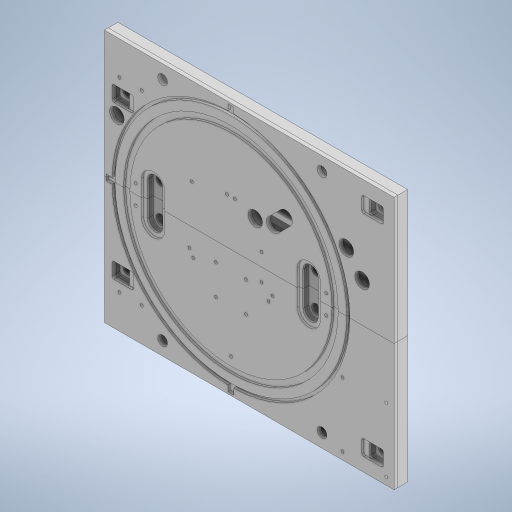
# Autodesk Inventor part: Корпус
Saved by Autodesk Inventor 2024 (Build 280153020, 153B)
## iProperties
Created: 2023-02-24
Part Number: Корпус
Material: Типовые
Document SubType Name: Modeling
Designer: Admin
Density: 1 g/cm^3
Appearance: По умолчанию
Author: Admin
Autodesk Inventor part; units mm, degrees
(part 1 of 3)
ref_plane "YZ Plane" through (0, 0, 0) normal (1, 0, 0) x (0, 1, 0)
ref_plane "XZ Plane" through (0, 0, 0) normal (0, 1, 0) x (-1, 0, 0)
ref_plane "XY Plane" through (0, 0, 0) normal (0, 0, 1) x (1, 0, 0)
sketch "Эскиз1" plane through (0, 0, 0) normal (0, 0, 1) x (1, 0, 0)
  circle A0 centre (0, 0) radius 118.266 construction
  circle A1 centre (0, 0) radius 119.25
  line L0 (-126.25, 126.25) -> (163.75, 126.25)
  line L1 (163.75, 126.25) -> (163.75, -126.25)
  line L2 (163.75, -126.25) -> (-126.25, -126.25)
  line L3 (-126.25, -126.25) -> (-126.25, 126.25)
  circle A2 centre (0, 0) radius 122.25
  line L4 (-3, 122.2132) -> (-3, 128.25)
  line L5 (-3, 128.25) -> (3, 128.25)
  line L6 (3, 128.25) -> (3, 122.2132)
  line L7 (-122.2132, 3) -> (-128.25, 3)
  line L8 (-128.25, 3) -> (-128.25, -3)
  line L9 (-128.25, -3) -> (-122.2132, -3)
  line L10 (3, -122.2132) -> (3, -128.25)
  line L11 (3, -128.25) -> (-3, -128.25)
  line L12 (-3, -128.25) -> (-3, -122.2132)
  line L13 (167.75, 130.25) -> (-130.25, 130.25)
  line L14 (-130.25, 130.25) -> (-130.25, -130.25)
  line L15 (-130.25, -130.25) -> (167.75, -130.25)
  line L16 (167.75, -130.25) -> (167.75, 130.25)
  line L17 (-126.25, 126.25) -> (-126.25, 130.25)
  line L18 (-126.25, -126.25) -> (-126.25, -130.25)
  line L19 (163.75, -126.25) -> (163.75, -130.25)
  line L20 (163.75, 126.25) -> (163.75, 130.25)
  circle A3 centre (0, 0) radius 104
  circle A4 centre (0, 0) radius 110.3675
  circle A5 centre (0, 0) radius 63
  line L21 (-80.25, 126.25) -> (-126.25, 126.25)
  line L22 (-80.25, 101.25) -> (-80.25, 126.25)
  line L23 (-126.25, 126.25) -> (-126.25, 101.25)
  line L24 (-126.25, 101.25) -> (-80.25, 101.25)
  line L25 (-126.25, -126.25) -> (-80.25, -126.25)
  line L26 (-80.25, -101.25) -> (-126.25, -101.25)
  line L27 (-126.25, -101.25) -> (-126.25, -126.25)
  line L28 (-80.25, -126.25) -> (-80.25, -101.25)
  line L29 (-70.25, 121.25) -> (93.75, 121.25) construction
  line L30 (-70.25, 111.25) -> (93.75, 111.25) construction
  circle A6 centre (93.75, 116.25) radius 5
  circle A7 centre (-70.25, 116.25) radius 5
  circle A8 centre (0, 0) radius 55.4255 construction
  line L31 (0, -27.1116) -> (0, -26.4367) construction
  line L32 (0, 0) -> (156.4435, 0) construction
  line L33 (0, 0) -> (156.0708, 16.4588) construction
  line L34 (0, 0) -> (155.7905, -16.4292) construction
  line L35 (-128.25, 0) -> (-119.25, 0)
  line L36 (0, -128.25) -> (0, -119.25)
  line L37 (0, 128.25) -> (0, 119.25)
  line L38 (163.75, 116.25) -> (163.75, 100.25)
  line L39 (163.75, 100.25) -> (163.75, 116.25)
  circle A9 centre (0, -34.641) radius 20.7845 construction
  line L40 (93, -126.25) -> (108, -126.25)
  line L41 (-76, -126.25) -> (-61, -126.25)
  line L42 (14, -6) -> (49, -6) construction
  line L43 (49, -6) -> (49, 6) construction
  line L44 (49, 6) -> (14, 6) construction
  line L45 (14, 6) -> (14, -6) construction
  line L46 (14, -6) -> (49, 6) construction
  line L47 (49, -6) -> (14, 6) construction
  line L48 (36.5689, 0.8398) -> (49, 2.1508) construction
  line L49 (49, 2.1508) -> (48.3707, 8.1177) construction
  line L50 (48.3707, 8.1177) -> (35.9397, 6.8067) construction
  line L51 (35.9397, 6.8067) -> (36.5689, 0.8398) construction
  line L52 (36.5689, 0.8398) -> (48.3707, 8.1177) construction
  line L53 (49, 2.1508) -> (35.9397, 6.8067) construction
  line L54 (35.9397, -6.8067) -> (48.3707, -8.1177) construction
  line L55 (48.3707, -8.1177) -> (49, -2.1508) construction
  line L56 (49, -2.1508) -> (36.5689, -0.8398) construction
  line L57 (36.5689, -0.8398) -> (35.9397, -6.8067) construction
  line L58 (35.9397, -6.8067) -> (49, -2.1508) construction
  line L59 (48.3707, -8.1177) -> (36.5689, -0.8398) construction
  line L60 (14, -11) -> (49, -11)
  line L61 (49, -11) -> (49, 11)
  line L62 (49, 11) -> (14, 11)
  line L63 (19, 11) -> (19, -11)
  line L64 (0, 0) -> (63, 0) construction
  line L65 (34.5, -11) -> (28.5, -11)
  line L66 (28.5, -11) -> (28.5, -16)
  line L67 (28.5, -16) -> (34.5, -16)
  line L68 (34.5, -16) -> (34.5, -11)
  line L69 (28.5, 11) -> (34.5, 11)
  line L70 (34.5, 11) -> (34.5, 16)
  line L71 (34.5, 16) -> (28.5, 16)
  line L72 (28.5, 16) -> (28.5, 11)
  circle A10 centre (31.5, 13.5) radius 1.5
  line L73 (29.9412, 10.8) -> (28.3823, 13.5)
  line L74 (28.3823, 13.5) -> (29.9412, 16.2)
  line L75 (29.9412, 16.2) -> (33.0588, 16.2)
  line L76 (33.0588, 16.2) -> (34.6177, 13.5)
  line L77 (34.6177, 13.5) -> (33.0588, 10.8)
  line L78 (33.0588, 10.8) -> (29.9412, 10.8)
  arc A11 (34.5, 16) -> (49, 11) centre (49, 34.525) ccw
  arc A12 (49, -11) -> (34.5, -16) centre (49, -34.525) ccw
  arc A13 (14, -11) -> (28.5, -16) centre (28.5, 7.525) ccw
  arc A14 (28.5, 16) -> (16.5, 9) centre (28.5, 2.2143) ccw construction
  circle A15 centre (93.75, -116.25) radius 5
  line L79 (-70.25, -111.25) -> (93.75, -111.25) construction
  line L80 (-70.25, -121.25) -> (93.75, -121.25) construction
  circle A16 centre (-70.25, -116.25) radius 5
  circle A17 centre (-117.25, 60.75) radius 7.5
  circle A18 centre (118.75, 60.75) radius 7.5
  line L81 (-117.25, 68.25) -> (118.75, 68.25) construction
  line L82 (118.75, 53.25) -> (-117.25, 53.25) construction
  circle A19 centre (25, 40) radius 7.5
  circle A20 centre (135, 40) radius 7.5
  line L83 (135, 47.5) -> (25, 47.5) construction
  line L84 (135, 32.5) -> (25, 32.5) construction
  line L85 (162.25, -54.75) -> (112.25, -54.75)
  line L86 (112.25, -54.75) -> (112.25, -124.75)
  line L87 (112.25, -124.75) -> (162.25, -124.75)
  line L88 (162.25, -124.75) -> (162.25, -54.75)
  circle A21 centre (159.75, -56.75) radius 1.5
  circle A22 centre (114.75, -56.75) radius 1.5
  circle A23 centre (114.75, -122.75) radius 1.5
  circle A24 centre (159.75, -122.75) radius 1.5
  line L89 (137.25, -89.75) -> (144.5274, -89.75) construction
  line L90 (144.5274, -89.75) -> (137.25, -89.75) construction
  line L91 (137.25, -89.75) -> (137.25, -87.3142) construction
  circle A25 centre (-47.6314, -27.5) radius 8 construction
  circle A26 centre (0, 55) radius 8 construction
  circle A27 centre (-47.6314, -27.5) radius 2.5
  line L92 (54.5596, -31.5) -> (0, 63) construction
  line L93 (0, 63) -> (-54.5596, -31.5) construction
  line L94 (-54.5596, -31.5) -> (54.5596, -31.5) construction
  line L95 (-35.6542, -29.2452) -> (-49.5106, -37.2452)
  line L96 (-49.5106, -37.2452) -> (-57.0106, -24.2548)
  line L97 (-57.0106, -24.2548) -> (-43.1542, -16.2548)
  line L98 (-40.4221, -16.9869) -> (-34.9221, -26.5131)
  line L99 (-33.9221, -28.2452) -> (-57.0106, -24.2548) construction
  line L100 (-49.5106, -37.2452) -> (-41.4221, -15.2548) construction
  line L101 (-47.6314, -27.5) -> (0, 0) construction
  circle A28 centre (-42.7032, -20.0359) radius 1.5
  line L102 (0, 0) -> (0, 14.3794) construction
  circle A29 centre (-38.7032, -26.9641) radius 1.5
  line L103 (21.15, -13.491) -> (-21.15, -13.491)
  line L104 (-21.15, -13.491) -> (-21.15, -55.791)
  line L105 (-21.15, -55.791) -> (21.15, -55.791)
  line L106 (21.15, -55.791) -> (21.15, -13.491)
  line L107 (21.15, -13.491) -> (-21.15, -55.791) construction
  line L108 (-21.15, -13.491) -> (21.15, -55.791) construction
  circle A30 centre (15.5, -50.141) radius 1.5
  line L109 (0, -34.641) -> (0, -31.0481)
  line L110 (0, -34.641) -> (5.9719, -34.641)
  circle A31 centre (-15.5, -50.141) radius 1.5
  circle A32 centre (-15.5, -19.141) radius 1.5
  circle A33 centre (15.5, -19.141) radius 1.5
  line L111 (16.5, -13.491) -> (21.15, -18.141)
  line L112 (-16.5, -13.491) -> (-21.15, -18.141)
  line L113 (14, 11) -> (14, -11)
  line L114 (19, -11) -> (19, 11)
  line L115 (-43.1542, -16.2548) -> (-40.4221, -16.9869)
  line L116 (-35.6542, -29.2452) -> (-34.9221, -26.5131)
  line L117 (34.9221, -26.5131) -> (40.4221, -16.9869)
  line L118 (35.6542, -29.2452) -> (34.9221, -26.5131)
  line L119 (49.5106, -37.2452) -> (35.6542, -29.2452)
  line L120 (57.0106, -24.2548) -> (49.5106, -37.2452)
  line L121 (43.1542, -16.2548) -> (57.0106, -24.2548)
  line L122 (43.1542, -16.2548) -> (40.4221, -16.9869)
  circle A34 centre (42.7032, -20.0359) radius 1.5
  circle A35 centre (38.7032, -26.9641) radius 1.5
  circle A36 centre (47.6314, -27.5) radius 2.5
  circle A37 centre (47.6314, -27.5) radius 8 construction
  line L123 (57.0106, -24.2548) -> (33.9221, -28.2452) construction
  line L124 (41.4221, -15.2548) -> (49.5106, -37.2452) construction
  line L125 (5.5, 43.5) -> (-5.5, 43.5)
  line L126 (7.5, 45.5) -> (5.5, 43.5)
  line L127 (7.5, 61.5) -> (7.5, 45.5)
  line L128 (-7.5, 61.5) -> (7.5, 61.5)
  line L129 (-7.5, 45.5) -> (-7.5, 61.5)
  line L130 (-7.5, 45.5) -> (-5.5, 43.5)
  circle A38 centre (-4, 47) radius 1.5
  circle A39 centre (4, 47) radius 1.5
  circle A40 centre (0, 55) radius 2.5
  circle A41 centre (0, 55) radius 8 construction
  line L131 (-7.5, 61.5) -> (7.5, 43.5) construction
  line L132 (-7.5, 43.5) -> (7.5, 61.5) construction
  line L133 (163.75, -116.25) -> (163.75, -100.25)
  line L134 (163.75, -100.25) -> (163.75, -116.25)
  line L135 (-109.3, 75.8921) -> (-114.25, 73.0342)
  line L136 (-114.25, 73.0342) -> (-119.2, 75.8921)
  line L137 (-119.2, 75.8921) -> (-119.2, 81.6079)
  line L138 (-119.2, 81.6079) -> (-114.25, 84.4658)
  line L139 (-114.25, 84.4658) -> (-109.3, 81.6079)
  line L140 (-109.3, 81.6079) -> (-109.3, 75.8921)
  line L141 (-120.25, 70.75) -> (-108.25, 70.75)
  line L142 (-106.25, 72.75) -> (-106.25, 84.75)
  line L143 (-108.25, 86.75) -> (-120.25, 86.75)
  line L144 (-122.25, 84.75) -> (-122.25, 72.75)
  line L145 (-122.25, 70.75) -> (-106.25, 86.75) construction
  line L146 (-106.25, 70.75) -> (-122.25, 86.75) construction
  arc A42 (-120.25, 86.75) -> (-122.25, 84.75) centre (-120.25, 84.75) ccw
  arc A43 (-108.25, 70.75) -> (-106.25, 72.75) centre (-108.25, 72.75) ccw
  arc A44 (-106.25, 84.75) -> (-108.25, 86.75) centre (-108.25, 84.75) ccw
  arc A45 (-122.25, 72.75) -> (-120.25, 70.75) centre (-120.25, 72.75) ccw
  line L147 (-109.3, -75.8921) -> (-114.25, -73.0342)
  line L148 (-114.25, -73.0342) -> (-119.2, -75.8921)
  line L149 (-119.2, -75.8921) -> (-119.2, -81.6079)
  line L150 (-119.2, -81.6079) -> (-114.25, -84.4658)
  line L151 (-114.25, -84.4658) -> (-109.3, -81.6079)
  line L152 (-109.3, -81.6079) -> (-109.3, -75.8921)
  line L153 (-120.25, -70.75) -> (-108.25, -70.75)
  line L154 (-106.25, -72.75) -> (-106.25, -84.75)
  line L155 (-108.25, -86.75) -> (-120.25, -86.75)
  line L156 (-122.25, -84.75) -> (-122.25, -72.75)
  line L157 (-122.25, -70.75) -> (-106.25, -86.75) construction
  line L158 (-106.25, -70.75) -> (-122.25, -86.75) construction
  arc A46 (-122.25, -84.75) -> (-120.25, -86.75) centre (-120.25, -84.75) ccw
  arc A47 (-106.25, -72.75) -> (-108.25, -70.75) centre (-108.25, -72.75) ccw
  arc A48 (-108.25, -86.75) -> (-106.25, -84.75) centre (-108.25, -84.75) ccw
  arc A49 (-120.25, -70.75) -> (-122.25, -72.75) centre (-120.25, -72.75) ccw
  line L159 (-126.25, 101.25) -> (-80.25, 101.25)
  circle A50 centre (-114.75, 95.75) radius 1.5
  circle A51 centre (-91.75, 95.75) radius 1.5
  line L160 (-112.05, 97.3088) -> (-112.05, 94.1912)
  line L161 (-112.05, 94.1912) -> (-114.75, 92.6323)
  line L162 (-114.75, 92.6323) -> (-117.45, 94.1912)
  line L163 (-117.45, 94.1912) -> (-117.45, 97.3088)
  line L164 (-117.45, 97.3088) -> (-114.75, 98.8677)
  line L165 (-114.75, 98.8677) -> (-112.05, 97.3088)
  line L166 (-91.75, 98.8677) -> (-89.05, 97.3088)
  line L167 (-89.05, 97.3088) -> (-89.05, 94.1912)
  line L168 (-89.05, 94.1912) -> (-91.75, 92.6323)
  line L169 (-91.75, 92.6323) -> (-94.45, 94.1912)
  line L170 (-94.45, 94.1912) -> (-94.45, 97.3088)
  line L171 (-94.45, 97.3088) -> (-91.75, 98.8677)
  line L172 (-117.5, 91) -> (-112, 91)
  line L173 (-110, 93) -> (-110, 98.5)
  line L174 (-112, 100.5) -> (-117.5, 100.5)
  line L175 (-119.5, 98.5) -> (-119.5, 93)
  line L176 (-119.5, 91) -> (-110, 100.5) construction
  line L177 (-110, 91) -> (-119.5, 100.5) construction
  line L178 (-89, 100.5) -> (-94.5, 100.5)
  line L179 (-96.5, 98.5) -> (-96.5, 93)
  line L180 (-94.5, 91) -> (-89, 91)
  line L181 (-87, 93) -> (-87, 98.5)
  line L182 (-87, 100.5) -> (-96.5, 91) construction
  line L183 (-96.5, 100.5) -> (-87, 91) construction
  arc A52 (-119.5, 93) -> (-117.5, 91) centre (-117.5, 93) ccw
  arc A53 (-117.5, 100.5) -> (-119.5, 98.5) centre (-117.5, 98.5) ccw
  arc A54 (-110, 98.5) -> (-112, 100.5) centre (-112, 98.5) ccw
  arc A55 (-112, 91) -> (-110, 93) centre (-112, 93) ccw
  arc A56 (-96.5, 93) -> (-94.5, 91) centre (-94.5, 93) ccw
  arc A57 (-94.5, 100.5) -> (-96.5, 98.5) centre (-94.5, 98.5) ccw
  arc A58 (-89, 91) -> (-87, 93) centre (-89, 93) ccw
  arc A59 (-87, 98.5) -> (-89, 100.5) centre (-89, 98.5) ccw
  line L184 (-126.25, -101.25) -> (-80.25, -101.25)
  line L185 (-80.25, -101.25) -> (-80.25, -100.25)
  line L186 (-90.25, -90.25) -> (-116.25, -90.25)
  circle A60 centre (-91.75, -95.75) radius 1.5
  line L187 (-91.75, -92.6323) -> (-89.05, -94.1912)
  line L188 (-89.05, -94.1912) -> (-89.05, -97.3088)
  line L189 (-89.05, -97.3088) -> (-91.75, -98.8677)
  line L190 (-91.75, -98.8677) -> (-94.45, -97.3088)
  line L191 (-94.45, -97.3088) -> (-94.45, -94.1912)
  line L192 (-94.45, -94.1912) -> (-91.75, -92.6323)
  line L193 (-94.5, -100.5) -> (-89, -100.5)
  line L194 (-87, -98.5) -> (-87, -93)
  line L195 (-89, -91) -> (-94.5, -91)
  line L196 (-96.5, -93) -> (-96.5, -98.5)
  line L197 (-96.5, -100.5) -> (-87, -91) construction
  line L198 (-87, -100.5) -> (-96.5, -91) construction
  arc A61 (-94.5, -91) -> (-96.5, -93) centre (-94.5, -93) ccw
  arc A62 (-89, -100.5) -> (-87, -98.5) centre (-89, -98.5) ccw
  arc A63 (-96.5, -98.5) -> (-94.5, -100.5) centre (-94.5, -98.5) ccw
  arc A64 (-87, -93) -> (-89, -91) centre (-89, -93) ccw
  line L199 (-117.5, -100.5) -> (-112, -100.5)
  line L200 (-110, -98.5) -> (-110, -93)
  line L201 (-112, -91) -> (-117.5, -91)
  line L202 (-119.5, -93) -> (-119.5, -98.5)
  line L203 (-119.5, -100.5) -> (-110, -91) construction
  line L204 (-110, -100.5) -> (-119.5, -91) construction
  circle A65 centre (-114.75, -95.75) radius 1.5
  line L205 (-112.05, -94.1912) -> (-112.05, -97.3088)
  line L206 (-112.05, -97.3088) -> (-114.75, -98.8677)
  line L207 (-114.75, -98.8677) -> (-117.45, -97.3088)
  line L208 (-117.45, -97.3088) -> (-117.45, -94.1912)
  line L209 (-117.45, -94.1912) -> (-114.75, -92.6323)
  line L210 (-114.75, -92.6323) -> (-112.05, -94.1912)
  line L211 (-126.25, -100.25) -> (-126.25, -101.25)
  arc A66 (-117.5, -91) -> (-119.5, -93) centre (-117.5, -93) ccw
  arc A67 (-110, -93) -> (-112, -91) centre (-112, -93) ccw
  arc A68 (-112, -100.5) -> (-110, -98.5) centre (-112, -98.5) ccw
  arc A69 (-119.5, -98.5) -> (-117.5, -100.5) centre (-117.5, -98.5) ccw
  line L212 (-108.25, 86.75) -> (-102.25, 86.75)
  line L213 (-100.25, 84.75) -> (-100.25, 72.75)
  line L214 (-102.25, 70.75) -> (-108.25, 70.75)
  line L215 (-108.25, 70.75) -> (-108.25, 86.75)
  line L216 (-108.25, -86.75) -> (-102.25, -86.75)
  line L217 (-100.25, -84.75) -> (-100.25, -72.75)
  line L218 (-102.25, -70.75) -> (-108.25, -70.75)
  line L219 (-108.25, -70.75) -> (-108.25, -86.75)
  circle A70 centre (-114.25, 78.75) radius 3
  circle A71 centre (-114.25, -78.75) radius 3
  line L220 (4, 50.1177) -> (6.7, 48.5588)
  line L221 (6.7, 48.5588) -> (6.7, 45.4412)
  line L222 (6.7, 45.4412) -> (4, 43.8823)
  line L223 (4, 43.8823) -> (1.3, 45.4412)
  line L224 (1.3, 45.4412) -> (1.3, 48.5588)
  line L225 (1.3, 48.5588) -> (4, 50.1177)
  line L226 (-7.7, 42.25) -> (7.7, 42.25)
  line L227 (9.7, 44.25) -> (9.7, 49.75)
  line L228 (7.7, 51.75) -> (-7.7, 51.75)
  line L229 (-9.7, 49.75) -> (-9.7, 44.25)
  arc A72 (-7.7, 51.75) -> (-9.7, 49.75) centre (-7.7, 49.75) ccw
  arc A73 (7.7, 42.25) -> (9.7, 44.25) centre (7.7, 44.25) ccw
  arc A74 (-9.7, 44.25) -> (-7.7, 42.25) centre (-7.7, 44.25) ccw
  arc A75 (9.7, 49.75) -> (7.7, 51.75) centre (7.7, 49.75) ccw
  line L230 (0, 42.25) -> (0, 44.9705) construction
  circle A76 centre (-4, 47) radius 1.5
  line L231 (-6.7, 45.4412) -> (-4, 43.8823)
  line L232 (-6.7, 48.5588) -> (-6.7, 45.4412)
  line L233 (-4, 43.8823) -> (-1.3, 45.4412)
  line L234 (-4, 50.1177) -> (-6.7, 48.5588)
  line L235 (-1.3, 45.4412) -> (-1.3, 48.5588)
  line L236 (-1.3, 48.5588) -> (-4, 50.1177)
  line L237 (-42.7032, -16.9182) -> (-40.0032, -18.4771)
  arc A77 (-40.4396, -14.4566) -> (-43.1716, -13.7246) centre (-42.1716, -15.4566) ccw
  line L238 (-36.5896, -21.125) -> (-38.9456, -22.4853) construction
  arc A78 (-40.9668, -32.5434) -> (-38.2348, -33.2754) centre (-39.2348, -31.5434) ccw
  line L239 (-38.2348, -33.2754) -> (-33.4716, -30.5254)
  line L240 (-38.7032, -30.0818) -> (-36.0032, -28.5229)
  arc A79 (-33.4716, -30.5254) -> (-32.7396, -27.7934) centre (-34.4716, -28.7934) ccw
  line L241 (-41.4032, -28.5229) -> (-38.7032, -30.0818)
  line L242 (-36.0032, -28.5229) -> (-36.0032, -25.4053)
  line L243 (-41.4032, -25.4053) -> (-41.4032, -28.5229)
  line L244 (-38.7032, -23.8464) -> (-41.4032, -25.4053)
  line L245 (-36.0032, -25.4053) -> (-38.7032, -23.8464)
  line L246 (-40.0032, -18.4771) -> (-40.0032, -21.5947)
  line L247 (-40.0032, -21.5947) -> (-42.7032, -23.1536)
  line L248 (-42.7032, -23.1536) -> (-45.4032, -21.5947)
  line L249 (-45.4032, -21.5947) -> (-45.4032, -18.4771)
  line L250 (-32.7396, -27.7934) -> (-40.4396, -14.4566)
  line L251 (-48.6668, -19.2066) -> (-40.9668, -32.5434)
  arc A80 (-47.9348, -16.4746) -> (-48.6668, -19.2066) centre (-46.9348, -18.2066) ccw
  line L252 (-43.1716, -13.7246) -> (-47.9348, -16.4746)
  line L253 (-45.4032, -18.4771) -> (-42.7032, -16.9182)
  line L254 (36.0032, -28.5229) -> (36.0032, -25.4053)
  arc A81 (32.7396, -27.7934) -> (33.4716, -30.5254) centre (34.4716, -28.7934) ccw
  line L255 (36.5896, -21.125) -> (38.9456, -22.4853) construction
  arc A82 (48.6668, -19.2066) -> (47.9348, -16.4746) centre (46.9348, -18.2066) ccw
  line L256 (47.9348, -16.4746) -> (43.1716, -13.7246)
  line L257 (45.4032, -18.4771) -> (42.7032, -16.9182)
  arc A83 (43.1716, -13.7246) -> (40.4396, -14.4566) centre (42.1716, -15.4566) ccw
  line L258 (45.4032, -21.5947) -> (45.4032, -18.4771)
  line L259 (42.7032, -16.9182) -> (40.0032, -18.4771)
  line L260 (42.7032, -23.1536) -> (45.4032, -21.5947)
  line L261 (40.0032, -21.5947) -> (42.7032, -23.1536)
  line L262 (40.0032, -18.4771) -> (40.0032, -21.5947)
  line L263 (36.0032, -25.4053) -> (38.7032, -23.8464)
  line L264 (38.7032, -23.8464) -> (41.4032, -25.4053)
  line L265 (41.4032, -25.4053) -> (41.4032, -28.5229)
  line L266 (41.4032, -28.5229) -> (38.7032, -30.0818)
  line L267 (40.4396, -14.4566) -> (32.7396, -27.7934)
  line L268 (40.9668, -32.5434) -> (48.6668, -19.2066)
  arc A84 (38.2348, -33.2754) -> (40.9668, -32.5434) centre (39.2348, -31.5434) ccw
  line L269 (33.4716, -30.5254) -> (38.2348, -33.2754)
  line L270 (38.7032, -30.0818) -> (36.0032, -28.5229)
  line L271 (37.5303, -23.4956) -> (25.475, -16.5355)
  line L272 (24.743, -13.8035) -> (28.3843, -7.4965)
  line L273 (31.1164, -6.7645) -> (43.1716, -13.7246)
  line L274 (43.1716, -13.7246) -> (37.5303, -23.4956)
  line L275 (37.5303, -23.4956) -> (29.3843, -5.7645) construction
  line L276 (23.743, -15.5355) -> (43.1716, -13.7246) construction
  arc A85 (24.743, -13.8035) -> (25.475, -16.5355) centre (26.475, -14.8035) ccw
  arc A86 (31.1164, -6.7645) -> (28.3843, -7.4965) centre (30.1164, -8.4965) ccw
  line L277 (28.75, 8.75) -> (34.25, 8.75)
  line L278 (36.25, 10.75) -> (36.25, 16.25)
  line L279 (34.25, 18.25) -> (28.75, 18.25)
  line L280 (26.75, 16.25) -> (26.75, 10.75)
  line L281 (26.75, 8.75) -> (36.25, 18.25) construction
  line L282 (36.25, 8.75) -> (26.75, 18.25) construction
  arc A87 (28.75, 18.25) -> (26.75, 16.25) centre (28.75, 16.25) ccw
  arc A88 (36.25, 16.25) -> (34.25, 18.25) centre (34.25, 16.25) ccw
  arc A89 (26.75, 10.75) -> (28.75, 8.75) centre (28.75, 10.75) ccw
  arc A90 (34.25, 8.75) -> (36.25, 10.75) centre (34.25, 10.75) ccw
  line L283 (15.5, -16.0233) -> (18.2, -17.5822)
  line L284 (18.2, -17.5822) -> (18.2, -20.6998)
  line L285 (18.2, -20.6998) -> (15.5, -22.2587)
  line L286 (15.5, -22.2587) -> (12.8, -20.6998)
  line L287 (12.8, -20.6998) -> (12.8, -17.5822)
  line L288 (12.8, -17.5822) -> (15.5, -16.0233)
  line L289 (12.75, -23.891) -> (18.25, -23.891)
  line L290 (20.25, -21.891) -> (20.25, -16.391)
  line L291 (18.25, -14.391) -> (12.75, -14.391)
  line L292 (10.75, -16.391) -> (10.75, -21.891)
  line L293 (10.75, -23.891) -> (20.25, -14.391) construction
  line L294 (20.25, -23.891) -> (10.75, -14.391) construction
  arc A91 (12.75, -14.391) -> (10.75, -16.391) centre (12.75, -16.391) ccw
  arc A92 (18.25, -23.891) -> (20.25, -21.891) centre (18.25, -21.891) ccw
  arc A93 (10.75, -21.891) -> (12.75, -23.891) centre (12.75, -21.891) ccw
  arc A94 (20.25, -16.391) -> (18.25, -14.391) centre (18.25, -16.391) ccw
  arc A95 (-18.25, -45.391) -> (-20.25, -47.391) centre (-18.25, -47.391) ccw
  line L295 (-18.2, -48.5822) -> (-15.5, -47.0233)
  line L296 (-18.2, -51.6998) -> (-18.2, -48.5822)
  line L297 (-20.25, -47.391) -> (-20.25, -52.891)
  line L298 (-12.75, -45.391) -> (-18.25, -45.391)
  line L299 (-15.5, -47.0233) -> (-12.8, -48.5822)
  line L300 (-15.5, -53.2587) -> (-18.2, -51.6998)
  arc A96 (-10.75, -47.391) -> (-12.75, -45.391) centre (-12.75, -47.391) ccw
  line L301 (-12.8, -48.5822) -> (-12.8, -51.6998)
  line L302 (-20.25, -54.891) -> (-10.75, -45.391) construction
  line L303 (-10.75, -54.891) -> (-20.25, -45.391) construction
  line L304 (-10.75, -52.891) -> (-10.75, -47.391)
  line L305 (-18.25, -54.891) -> (-12.75, -54.891)
  line L306 (-12.8, -51.6998) -> (-15.5, -53.2587)
  arc A97 (-12.75, -54.891) -> (-10.75, -52.891) centre (-12.75, -52.891) ccw
  arc A98 (-20.25, -52.891) -> (-18.25, -54.891) centre (-18.25, -52.891) ccw
  arc A99 (12.75, -45.391) -> (10.75, -47.391) centre (12.75, -47.391) ccw
  line L307 (12.8, -48.5822) -> (15.5, -47.0233)
  line L308 (12.8, -51.6998) -> (12.8, -48.5822)
  line L309 (10.75, -47.391) -> (10.75, -52.891)
  line L310 (18.25, -45.391) -> (12.75, -45.391)
  line L311 (15.5, -47.0233) -> (18.2, -48.5822)
  line L312 (15.5, -53.2587) -> (12.8, -51.6998)
  arc A100 (20.25, -47.391) -> (18.25, -45.391) centre (18.25, -47.391) ccw
  line L313 (18.2, -48.5822) -> (18.2, -51.6998)
  line L314 (10.75, -54.891) -> (20.25, -45.391) construction
  line L315 (20.25, -54.891) -> (10.75, -45.391) construction
  line L316 (20.25, -52.891) -> (20.25, -47.391)
  line L317 (12.75, -54.891) -> (18.25, -54.891)
  line L318 (18.2, -51.6998) -> (15.5, -53.2587)
  arc A101 (18.25, -54.891) -> (20.25, -52.891) centre (18.25, -52.891) ccw
  arc A102 (10.75, -52.891) -> (12.75, -54.891) centre (12.75, -52.891) ccw
  arc A103 (-18.25, -14.391) -> (-20.25, -16.391) centre (-18.25, -16.391) ccw
  line L319 (-18.2, -17.5822) -> (-15.5, -16.0233)
  line L320 (-18.2, -20.6998) -> (-18.2, -17.5822)
  line L321 (-20.25, -16.391) -> (-20.25, -21.891)
  line L322 (-12.75, -14.391) -> (-18.25, -14.391)
  line L323 (-15.5, -16.0233) -> (-12.8, -17.5822)
  line L324 (-15.5, -22.2587) -> (-18.2, -20.6998)
  arc A104 (-10.75, -16.391) -> (-12.75, -14.391) centre (-12.75, -16.391) ccw
  line L325 (-12.8, -17.5822) -> (-12.8, -20.6998)
  line L326 (-20.25, -23.891) -> (-10.75, -14.391) construction
  line L327 (-10.75, -23.891) -> (-20.25, -14.391) construction
  line L328 (-10.75, -21.891) -> (-10.75, -16.391)
  line L329 (-18.25, -23.891) -> (-12.75, -23.891)
  line L330 (-12.8, -20.6998) -> (-15.5, -22.2587)
  arc A105 (-12.75, -23.891) -> (-10.75, -21.891) centre (-12.75, -21.891) ccw
  arc A106 (-20.25, -21.891) -> (-18.25, -23.891) centre (-18.25, -21.891) ccw
  circle A107 centre (-114.25, 78.75) radius 5.11
  circle A108 centre (-114.25, -78.75) radius 5.11
  arc A109 (-100.25, 84.75) -> (-102.25, 86.75) centre (-102.25, 84.75) ccw
  arc A110 (-102.25, 70.75) -> (-100.25, 72.75) centre (-102.25, 72.75) ccw
  arc A111 (-100.25, -72.75) -> (-102.25, -70.75) centre (-102.25, -72.75) ccw
  arc A112 (-102.25, -86.75) -> (-100.25, -84.75) centre (-102.25, -84.75) ccw
  arc A113 (-80.25, -100.25) -> (-90.25, -90.25) centre (-90.25, -100.25) ccw
  arc A114 (-116.25, -90.25) -> (-126.25, -100.25) centre (-116.25, -100.25) ccw
  line L331 (-80.25, 101.25) -> (-80.25, 100.25)
  line L332 (-90.25, 90.25) -> (-116.25, 90.25)
  arc A115 (-90.25, 90.25) -> (-80.25, 100.25) centre (-90.25, 100.25) ccw
  line L333 (-126.25, 101.25) -> (-126.25, 100.25)
  arc A116 (-126.25, 100.25) -> (-116.25, 90.25) centre (-116.25, 100.25) ccw
  line L334 (154.75, 100.25) -> (142.75, 100.25)
  line L335 (140.75, 100.25) -> (140.75, 114.25)
  line L336 (142.75, 116.25) -> (154.75, 116.25)
  line L337 (156.75, 114.25) -> (156.75, 102.25)
  line L338 (140.75, 116.25) -> (136.75, 116.25)
  line L339 (134.75, 114.25) -> (134.75, 102.25)
  line L340 (136.75, 100.25) -> (140.75, 100.25)
  line L341 (140.75, 102.25) -> (140.75, 116.25)
  circle A117 centre (148.75, 108.25) radius 3
  line L342 (145.8921, 103.3) -> (143.0342, 108.25)
  line L343 (143.0342, 108.25) -> (145.8921, 113.2)
  line L344 (145.8921, 113.2) -> (151.6079, 113.2)
  line L345 (151.6079, 113.2) -> (154.4658, 108.25)
  line L346 (154.4658, 108.25) -> (151.6079, 103.3)
  line L347 (151.6079, 103.3) -> (145.8921, 103.3)
  arc A118 (134.75, 102.25) -> (136.75, 100.25) centre (136.75, 102.25) ccw
  arc A119 (136.75, 116.25) -> (134.75, 114.25) centre (136.75, 114.25) ccw
  arc A120 (142.75, 116.25) -> (140.75, 114.25) centre (142.75, 114.25) ccw
  arc A121 (140.75, 102.25) -> (142.75, 100.25) centre (142.75, 102.25) ccw
  arc A122 (154.75, 100.25) -> (156.75, 102.25) centre (154.75, 102.25) ccw
  arc A123 (156.75, 114.25) -> (154.75, 116.25) centre (154.75, 114.25) ccw
  line L348 (142.75, 100.25) -> (140.75, 100.25)
  line L349 (142.75, 116.25) -> (140.75, 116.25)
  line L350 (154.75, -100.25) -> (142.75, -100.25)
  line L351 (140.75, -100.25) -> (140.75, -114.25)
  line L352 (142.75, -116.25) -> (154.75, -116.25)
  line L353 (156.75, -114.25) -> (156.75, -102.25)
  line L354 (140.75, -116.25) -> (136.75, -116.25)
  line L355 (134.75, -114.25) -> (134.75, -102.25)
  line L356 (136.75, -100.25) -> (140.75, -100.25)
  line L357 (140.75, -102.25) -> (140.75, -116.25)
  circle A124 centre (148.75, -108.25) radius 3
  line L358 (145.8921, -103.3) -> (143.0342, -108.25)
  line L359 (143.0342, -108.25) -> (145.8921, -113.2)
  line L360 (145.8921, -113.2) -> (151.6079, -113.2)
  line L361 (151.6079, -113.2) -> (154.4658, -108.25)
  line L362 (154.4658, -108.25) -> (151.6079, -103.3)
  line L363 (151.6079, -103.3) -> (145.8921, -103.3)
  arc A125 (136.75, -100.25) -> (134.75, -102.25) centre (136.75, -102.25) ccw
  arc A126 (134.75, -114.25) -> (136.75, -116.25) centre (136.75, -114.25) ccw
  arc A127 (140.75, -114.25) -> (142.75, -116.25) centre (142.75, -114.25) ccw
  arc A128 (142.75, -100.25) -> (140.75, -102.25) centre (142.75, -102.25) ccw
  arc A129 (156.75, -102.25) -> (154.75, -100.25) centre (154.75, -102.25) ccw
  arc A130 (154.75, -116.25) -> (156.75, -114.25) centre (154.75, -114.25) ccw
  line L364 (142.75, -100.25) -> (140.75, -100.25)
  line L365 (142.75, -116.25) -> (140.75, -116.25)
  circle A131 centre (148.75, -108.25) radius 5.11
  circle A132 centre (148.75, 108.25) radius 5.11
  arc A133 (28.5, 16) -> (14, 11) centre (28.5, -7.525) ccw
  circle A134 centre (31.5, -13.5) radius 1.5
  line L366 (31.5, -13.5) -> (40.351, -18.6101) construction
  line L367 (28.3823, -13.5) -> (29.9412, -10.8)
  line L368 (29.9412, -10.8) -> (33.0588, -10.8)
  line L369 (33.0588, -10.8) -> (34.6177, -13.5)
  line L370 (34.6177, -13.5) -> (33.0588, -16.2)
  line L371 (33.0588, -16.2) -> (29.9412, -16.2)
  line L372 (29.9412, -16.2) -> (28.3823, -13.5)
  point P0 (0, 122.25)
  point P1 (0, -122.25)
  point P2 (-122.25, 0)
  point P3 (42.4698, 4.4787)
  point P4 (42.4698, -4.4787)
  point P5 (31.5, 0)
  point P6 (31.5, -11)
  point P7 (28.5, 13.5)
  point P8 (112.25, -89.75)
  point P9 (137.25, -124.75)
  point P10 (-45.4663, -26.25)
  point P11 (-45.4663, -26.25)
  point P12 (54.5596, -31.5)
  point P13 (45.4663, -26.25)
  point P14 (0, 63)
  point P15 (0, 52.5)
  point P16 (-126.25, 95.75)
  point P17 (-100.25, 86.75)
  point P18 (-100.25, -70.75)
  point P19 (-9.7, 47)
  point P20 (-35.8532, -31.9004)
  point P21 (-38.7032, -26.9641)
  point P22 (-38.7032, -26.9641)
  point P23 (-42.7032, -20.0359)
  point P24 (-38.7032, -26.9641)
  point P25 (-42.7032, -20.0359)
  point P26 (45.5532, -15.0996)
  point P27 (42.7032, -20.0359)
  point P28 (42.7032, -20.0359)
  point P29 (38.7032, -26.9641)
  point P30 (42.7032, -20.0359)
  point P31 (38.7032, -26.9641)
  point P32 (35.7982, -22.4956)
  point P33 (-108.25, -70.75)
  point P34 (-80.25, 90.25)
  point P35 (-126.25, 90.25)
  point P36 (156.75, 108.25)
  point P37 (148.75, 100.25)
  point P38 (156.75, -108.25)
  point P39 (148.75, -100.25)
  point P40 (153.6712, -109.6263)
  point P41 (152.4025, -111.8237)
  point P42 (150.0187, -113.2)
  point P43 (147.4813, -113.2)
  point P44 (152.4025, -104.6763)
  point P45 (153.6712, -106.8737)
  point P46 (145.0975, -111.8237)
  point P47 (143.8288, -109.6263)
  point P48 (147.4813, -103.3)
  point P49 (150.0187, -103.3)
  point P50 (143.8288, -106.8737)
  point P51 (145.0975, -104.6763)
  point P52 (31.5, 11)
  point P53 (31.5, 11)
  point P54 (31.5, -11)
  point P55 (40.351, -18.6101)
  point P56 (34.5, -13.5)
  dimension "d2" = 236.532
  dimension "d3" = 238.5
  dimension "d4" = 290
  dimension "d5" = 3
  dimension "d6" = 6
  dimension "d7" = 4
  dimension "d8" = 208
  dimension "d9" = 220.735
  dimension "d10" = 126
  dimension "d11" = 4
  dimension "d12" = 2
  dimension "d13" = 2
  dimension "d14" = 2
  dimension "d15" = 25
  dimension "d16" = 46
  dimension "d17" = 25
  dimension "d21" = 10
  dimension "d22" = 10
  dimension "d27" = 110.851
  dimension "d28" = 6.02
  dimension "d29" = 6.02
  dimension "d40" = 41.569
  dimension "d56" = 12
  dimension "d57" = 35
  dimension "d58" = 6
  dimension "d59" = 12.5
  dimension "d60" = 5
  dimension "d63" = 5
  dimension "d64" = 6
  dimension "d66" = 10
  dimension "d67" = 10
  dimension "d69" = 58
  dimension "d71" = 45
  dimension "d72" = 15
  dimension "d73" = 40
  dimension "d74" = 25
  dimension "d75" = 15
  dimension "d76" = 110
  dimension "d77" = 70
  dimension "d78" = 50
  dimension "d80" = 63
  dimension "d81" = 3
  dimension "d82" = 1.5
  dimension "d114" = 4
  dimension "d115" = 18
  dimension "d116" = 15
  dimension "d117" = 3
  dimension "d118" = 2
  dimension "d119" = 2
  dimension "d120" = 5
  dimension "d122" = 236
  dimension "d123" = 42.3
  dimension "d125" = 31
  dimension "d126" = 31
  dimension "d129" = 33
  dimension "d131" = 30
  dimension "d132" = 5
  dimension "d133" = 22
  dimension "d134" = 2
  dimension "d135" = 2
  dimension "d136" = 2
  dimension "d137" = 2
  dimension "d140" = 360
  dimension "d144" = 1.5
  constraints: 750 end point, 181 point on circle, 148 point on line, 138 tangent, 130 centre point, 72 symmetric about line, 61 parallel, 50 midpoint, 48 equal radius, 47 perpendicular, 40 coincident, 37 horizontal, 25 equal length, 25 vertical alignment, 19 vertical, 15 horizontal alignment, 3 collinear, 454 other
  measures "d2" diameter of A0
  measures "d3" diameter of A1
  measures "d4" distance of L3.end L0.end
  measures "d6" distance between parallel lines of L4 L6
  measures "d7" distance between parallel lines of L0 L13
  measures "d8" diameter of A3
  measures "d9" diameter of A4
  measures "d10" diameter of A5
  measures "d11" distance from line of point (-122.25, 0) L3
  measures "d12" distance between parallel lines of L0 L5
  measures "d13" distance between parallel lines of L3 L8
  measures "d14" distance between parallel lines of L2 L11
  measures "d15" distance of L3.end L24.start
  measures "d16" distance of L3.end L21.start
  measures "d17" distance of L3.start L26.end
  measures "d21" diameter of A7
  measures "d22" diameter of A6
  measures "d27" diameter of A8
  measures "d28" angle of L32 L33
  measures "d29" angle of L32 L34
  measures "d40" diameter of A9
  measures "d56" distance of L42.end L44.start
  measures "d57" distance of L44.start L44.end
  measures "d58" distance of L49.start L50.start
  measures "d59" distance of L50.start L50.end
  measures "d60" distance between parallel lines of L44 L62
  measures "d63" distance of L65.end L67.start
  measures "d64" distance of L67.start L67.end
  measures "d66" distance from line of L22 A7.centre
  measures "d67" distance from line of L0 A7.centre
  measures "d69" distance between parallel lines of L0 L81
  measures "d71" distance from line of L1 A18.centre
  measures "d72" diameter of A19
  measures "d73" vertical distance of A3.centre A19.centre
  measures "d74" horizontal distance of A3.centre A19.centre
  measures "d75" diameter of A20
  measures "d76" distance of L84.start L84.end
  measures "d77" distance of L88.start L88.end
  measures "d78" distance of L88.end L86.start
  measures "d81" diameter of A23
  measures "d82" distance between parallel lines of L2 L87
  measures "d114" distance edge to line of A27 L96
  measures "d115" distance of L96.end L100.end
  measures "d116" distance of L100.end L99.start
  measures "d117" diameter of A28
  measures "d118" distance edge to line of A28 L98
  measures "d119" distance edge to line of A28 L97
  measures "d120" diameter of A27
  measures "d122" distance of L81.start L81.end
  measures "d123" distance of L104.end L105.end
  measures "d125" distance of A33.centre A30.centre
  measures "d126" distance of A32.centre A33.centre
  measures "d129" distance of L112.start L111.start
  measures "d131" distance between parallel lines of L63 L61
  measures "d132" distance between parallel lines of L113 L63
  measures "d133" distance of L60.end L62.start
  measures "d134" distance of L97.end L100.end
  measures "d135" distance of L98.start L100.end
  measures "d136" distance of L95.start L99.start
  measures "d137" distance of L98.end L99.start
  measures "d144" distance between parallel lines of L1 L88
extrude "Выдавливание1" add sketch "Эскиз1" against normal blind 10 contours A1 | A1 L37 A2 L36 | A1 L35 A2 L37 | L36 A2 L35 A1 | L37 L0 L6 A2 | A2 L4 L0 L37 | L36 L2 L12 A2 | A2 L10 L2 L36 | L35 L3 L7 A2 | A2 L9 L3 L35 | L6 L0 L1 L2 L10 A2 | A2 L7 L3 A116 L332 A115 L331 L22 L0 L4 | L37 L5 L6 L0 | L0 L4 L5 L37 | L12 L2 L28 L185 A113 L186 A114 L3 L9 A2 | L36 L11 L12 L2 | L2 L10 L11 L36 | L35 L8 L7 L3 | L3 L9 L8 L35 | L6 L5 L4 L0 L17 L13 L20 | L12 L11 L10 L2 L19 L15 L18 | L7 L8 L9 L3 L18 L15 L14 L13 L17 | L20 L13 L16 L15 L19 L1 | L22 L24 L3 L0 | L3 L24 L331 A115 L332 A116 | A114 L186 A113 L185 L26 L3 | L26 L28 L2 L3 | A3 | A4 | A5 | A6 | A7 | L113 L62 L63 L60 | L60 L272 A85 A13 L106 L103 | L63 L62 L280 A89 L277 A90 L278 L61 L60 L273 A86 L272 | L103 L106 A13 | A13 L106 L111 L290 A94 L291 L103 | A133 L280 L62 | L272 A86 L273 L60 L369 L368 L367 | L60 L66 L367 L372 A13 A85 L272 | L111 L291 A91 L292 A93 L289 A92 L290 L106 L105 L104 L112 L321 A106 L329 A105 L328 A104 L322 L103 | A133 L72 L74 L73 L62 L280 | L280 A87 L279 A88 L278 A11 L71 L76 L75 L74 A133 | L60 L367 L66 | L62 L73 L78 L77 L278 A90 L277 A89 L280 | A13 L67 L372 L371 L370 A12 L273 A83 L267 L271 A85 | L112 L322 A103 L321 L104 L103 | L291 A94 L290 L111 | L111 L290 A92 L289 A93 L292 A91 L291 | L71 L74 L72 | L367 L368 L369 L60 | L60 L369 L68 L370 L67 L372 L66 L367 | L66 L372 L367 | L72 L73 L62 | L66 L372 L67 | L322 A104 L328 A105 L329 A106 L321 L112 | L112 L321 A103 L322 | L74 L75 L76 L71 | L71 L76 L70 L77 L62 L73 L72 L74 | L72 L73 L74 | L60 L68 L369 | L273 A12 L68 L370 L369 L60 | L60 A12 L273 | L62 L77 L78 L73 | L67 L370 L371 L372 | L271 L117 L118 L119 L268 A84 L269 A81 L267 | L267 A83 L274 L122 L117 L271 | L71 L70 L76 | L369 L370 L68 | L77 L70 L62 | L370 L68 L67 | L271 L274 L262 L261 L260 L258 L257 L259 L122 L121 L268 L119 L118 L117 | L117 L122 L274 L259 L262 L271 | A11 L278 L62 L70 L77 L76 | L76 L77 L70 | L62 L278 A11 | L256 A82 L268 L121 L122 L274 | L274 L259 L257 L258 L260 L261 L262 | L262 L259 L274 | L268 L121 L120 L119 | A10 | A15 | A16 | A17 | A18 | A19 | A20 | L88 L87 L86 L85 | A21 | A22 | A23 | A24 | A27 | L116 L98 L115 L97 L251 A80 L252 A77 L250 A79 L239 A78 L95 | L95 L251 L97 L115 L98 L116 | L95 L96 L97 L251 | A28 | A29 | A30 | A31 | A32 | A33 | A34 | A35 | A36 | L126 L127 L228 A75 L227 A73 L226 A74 L229 A72 L129 L130 L125 | L125 L130 L129 L228 L127 L126 | L228 L129 L128 L127 | A38 | A39 | A40 | L135 A107 L140 | A107 L135 | L135 A107 L136 L137 L138 L139 L140 | L140 A107 | L135 L136 A107 | A107 L139 L140 | A107 L136 | L139 A107 | L136 L137 A107 | A107 L138 L139 | A107 L137 | L138 A107 | L137 L138 A107 | A45 L144 A42 L143 L215 L141 | L215 A44 L142 A43 | A43 L142 A44 L212 A109 L213 A110 L214 | L152 A108 L147 | A108 L152 L151 L150 L149 L148 L147 | L147 A108 | A108 L152 | A108 L148 L147 | L152 L151 A108 | L148 A108 | A108 L151 | A108 L149 L148 | L151 L150 A108 | L149 A108 | A108 L150 | A108 L150 L149 | L153 L219 L155 A46 L156 A49 | L218 A111 L217 A112 L216 A48 L154 A47 | A47 L154 A48 L219 | A50 | A51 | L160 L161 L162 L163 L164 L165 | L166 L167 L168 L169 L170 L171 | A52 L175 A53 L174 A54 L173 A55 L172 | A59 L181 A58 L180 A56 L179 A57 L178 | A60 | L187 L188 L189 L190 L191 L192 | A63 L196 A61 L195 A64 L194 A62 L193 | A69 L202 A66 L201 A67 L200 A68 L199 | A65 | L205 L206 L207 L208 L209 L210 | A70 | A71 | L220 L221 L222 L223 L224 L225 | L232 L234 L236 L235 L233 L231 | L237 L246 L247 L248 L249 L253 | L241 L243 L244 L245 L242 L240 | L254 L263 L264 L265 L266 L270 | L283 L284 L285 L286 L287 L288 | L298 A96 L304 A97 L305 A98 L297 A95 | L295 L299 L301 L306 L300 L296 | L310 A100 L316 A101 L317 A102 L309 A99 | L307 L311 L313 L318 L312 L308 | L319 L323 L325 L330 L324 L320 | L334 A121 L335 A120 L336 A123 L337 A122 | L348 L335 A121 | L335 L340 A118 L339 A119 L338 L341 | L341 L349 A120 | A117 | L342 A132 L347 | A132 L342 | L342 A132 L343 L344 L345 L346 L347 | L347 A132 | L342 L343 A132 | A132 L346 L347 | A132 L343 | L346 A132 | L343 L344 A132 | A132 L345 L346 | A132 L344 | L344 L345 A132 | L345 A132 | A129 L353 A130 L352 A127 L351 A128 L350 | A128 L351 L364 | L351 L357 L354 A126 L355 A125 L356 | A127 L365 L357 | A124 | L363 A131 L358 | A131 L363 L362 L361 L360 L359 L358 | L358 A131 | A131 L363 | A131 L359 L358 | L363 L362 A131 | L359 A131 | A131 L362 | A131 L360 L359 | L362 L361 A131 | L360 A131 | A131 L361 L360 | A131 L361 | A134
sketch "Эскиз2" plane through (0, 0, 0) normal (0, 0, 1) x (1, 0, 0)
  line L0 (-70.25, -111.25) -> (93.75, -111.25) projected
  line L1 (-70.25, -121.25) -> (93.75, -121.25) projected
  circle A0 centre (93.75, -116.25) radius 5 projected
  circle A1 centre (-70.25, -116.25) radius 5 projected
  circle A2 centre (-117.25, 60.75) radius 7.5 projected
  line L2 (-117.25, 68.25) -> (118.75, 68.25) projected
  line L3 (118.75, 53.25) -> (-117.25, 53.25) projected
  circle A3 centre (118.75, 60.75) radius 7.5 projected
  line L4 (-70.25, 111.25) -> (93.75, 111.25) projected
  circle A4 centre (93.75, 116.25) radius 5 projected
  line L5 (-70.25, 121.25) -> (93.75, 121.25) projected
  circle A5 centre (-70.25, 116.25) radius 5 projected
  line L6 (135, 47.5) -> (25, 47.5) projected
  line L7 (135, 32.5) -> (25, 32.5) projected
  circle A6 centre (135, 40) radius 7.5 projected
  circle A7 centre (25, 40) radius 7.5 projected
  line L8 (163.75, 0) -> (122.5, 0) construction
  line L9 (-80, -17.5) -> (-80, 17.5)
  line L10 (-89.95, -17.5) -> (-89.95, 17.5)
  line L11 (-70.05, 17.5) -> (-70.05, -17.5)
  arc A8 (-89.95, -17.5) -> (-70.05, -17.5) centre (-80, -17.5) ccw
  arc A9 (-70.05, 17.5) -> (-89.95, 17.5) centre (-80, 17.5) ccw
  circle A10 centre (-80, 17.5) radius 3
  line L12 (0, 0) -> (0, 19.2285) construction
  line L13 (-75.05, 20.3579) -> (-75.05, 14.6421)
  line L14 (-75.05, 14.6421) -> (-80, 11.7842)
  line L15 (-80, 11.7842) -> (-84.95, 14.6421)
  line L16 (-84.95, 14.6421) -> (-84.95, 20.3579)
  line L17 (-84.95, 20.3579) -> (-80, 23.2158)
  line L18 (-80, 23.2158) -> (-75.05, 20.3579)
  circle A11 centre (-80, -17.5) radius 3
  circle A12 centre (-80, 17.5) radius 5.11
  circle A13 centre (-80, -17.5) radius 5.11
  line L19 (-72.05, -17.5) -> (-72.05, 17.5)
  arc A14 (-72.05, 17.5) -> (-87.95, 17.5) centre (-80, 17.5) ccw
  line L20 (-87.95, 17.5) -> (-87.95, -17.5)
  arc A15 (-87.95, -17.5) -> (-72.05, -17.5) centre (-80, -17.5) ccw
  line L21 (-75.05, -14.6421) -> (-75.05, -20.3579)
  line L22 (-75.05, -20.3579) -> (-80, -23.2158)
  line L23 (-80, -23.2158) -> (-84.95, -20.3579)
  line L24 (-84.95, -20.3579) -> (-84.95, -14.6421)
  line L25 (-84.95, -14.6421) -> (-80, -11.7842)
  line L26 (-80, -11.7842) -> (-75.05, -14.6421)
  circle A16 centre (80, -17.5) radius 3
  line L27 (80, 23.2158) -> (75.05, 20.3579)
  arc A17 (89.95, 17.5) -> (70.05, 17.5) centre (80, 17.5) ccw
  line L28 (75.05, 20.3579) -> (75.05, 14.6421)
  arc A18 (87.95, 17.5) -> (72.05, 17.5) centre (80, 17.5) ccw
  line L29 (75.05, 14.6421) -> (80, 11.7842)
  circle A19 centre (80, 17.5) radius 3
  circle A20 centre (80, 17.5) radius 5.11
  line L30 (84.95, 14.6421) -> (84.95, 20.3579)
  line L31 (80, 11.7842) -> (84.95, 14.6421)
  line L32 (84.95, 20.3579) -> (80, 23.2158)
  line L33 (89.95, -17.5) -> (89.95, 17.5)
  line L34 (87.95, 17.5) -> (87.95, -17.5)
  line L35 (80, -17.5) -> (80, 17.5)
  line L36 (72.05, -17.5) -> (72.05, 17.5)
  line L37 (70.05, 17.5) -> (70.05, -17.5)
  arc A21 (70.05, -17.5) -> (89.95, -17.5) centre (80, -17.5) ccw
  circle A22 centre (80, -17.5) radius 5.11
  arc A23 (72.05, -17.5) -> (87.95, -17.5) centre (80, -17.5) ccw
  line L38 (75.05, -14.6421) -> (75.05, -20.3579)
  line L39 (75.05, -20.3579) -> (80, -23.2158)
  line L40 (80, -23.2158) -> (84.95, -20.3579)
  line L41 (84.95, -20.3579) -> (84.95, -14.6421)
  line L42 (84.95, -14.6421) -> (80, -11.7842)
  line L43 (80, -11.7842) -> (75.05, -14.6421)
  circle A24 centre (114.75, -122.75) radius 1.5 projected
  circle A25 centre (114.75, -56.75) radius 1.5 projected
  circle A26 centre (159.75, -56.75) radius 1.5 projected
  circle A27 centre (159.75, -122.75) radius 1.5 projected
  line L44 (157, -118) -> (162.5, -118)
  line L45 (164.5, -120) -> (164.5, -125.5)
  line L46 (162.5, -127.5) -> (157, -127.5)
  line L47 (155, -125.5) -> (155, -120)
  line L48 (155, -118) -> (164.5, -127.5) construction
  line L49 (164.5, -118) -> (155, -127.5) construction
  line L50 (112, -118) -> (117.5, -118)
  line L51 (119.5, -120) -> (119.5, -125.5)
  line L52 (117.5, -127.5) -> (112, -127.5)
  line L53 (110, -125.5) -> (110, -120)
  line L54 (110, -118) -> (119.5, -127.5) construction
  line L55 (119.5, -118) -> (110, -127.5) construction
  line L56 (112, -52) -> (117.5, -52)
  line L57 (119.5, -54) -> (119.5, -59.5)
  line L58 (117.5, -61.5) -> (112, -61.5)
  line L59 (110, -59.5) -> (110, -54)
  line L60 (110, -52) -> (119.5, -61.5) construction
  line L61 (119.5, -52) -> (110, -61.5) construction
  line L62 (157, -52) -> (162.5, -52)
  line L63 (164.5, -54) -> (164.5, -59.5)
  line L64 (162.5, -61.5) -> (157, -61.5)
  line L65 (155, -59.5) -> (155, -54)
  line L66 (155, -52) -> (164.5, -61.5) construction
  line L67 (164.5, -52) -> (155, -61.5) construction
  line L68 (162.45, -121.1912) -> (162.45, -124.3088)
  line L69 (162.45, -124.3088) -> (159.75, -125.8677)
  line L70 (159.75, -125.8677) -> (157.05, -124.3088)
  line L71 (157.05, -124.3088) -> (157.05, -121.1912)
  line L72 (157.05, -121.1912) -> (159.75, -119.6323)
  line L73 (159.75, -119.6323) -> (162.45, -121.1912)
  arc A28 (155, -125.5) -> (157, -127.5) centre (157, -125.5) ccw
  arc A29 (164.5, -120) -> (162.5, -118) centre (162.5, -120) ccw
  arc A30 (157, -118) -> (155, -120) centre (157, -120) ccw
  arc A31 (162.5, -127.5) -> (164.5, -125.5) centre (162.5, -125.5) ccw
  arc A32 (110, -125.5) -> (112, -127.5) centre (112, -125.5) ccw
  arc A33 (112, -118) -> (110, -120) centre (112, -120) ccw
  arc A34 (119.5, -120) -> (117.5, -118) centre (117.5, -120) ccw
  arc A35 (117.5, -127.5) -> (119.5, -125.5) centre (117.5, -125.5) ccw
  arc A36 (119.5, -54) -> (117.5, -52) centre (117.5, -54) ccw
  arc A37 (117.5, -61.5) -> (119.5, -59.5) centre (117.5, -59.5) ccw
  arc A38 (110, -59.5) -> (112, -61.5) centre (112, -59.5) ccw
  arc A39 (112, -52) -> (110, -54) centre (112, -54) ccw
  arc A40 (164.5, -54) -> (162.5, -52) centre (162.5, -54) ccw
  arc A41 (162.5, -61.5) -> (164.5, -59.5) centre (162.5, -59.5) ccw
  arc A42 (155, -59.5) -> (157, -61.5) centre (157, -59.5) ccw
  arc A43 (157, -52) -> (155, -54) centre (157, -54) ccw
  line L74 (117.45, -121.1912) -> (117.45, -124.3088)
  line L75 (117.45, -124.3088) -> (114.75, -125.8677)
  line L76 (114.75, -125.8677) -> (112.05, -124.3088)
  line L77 (112.05, -124.3088) -> (112.05, -121.1912)
  line L78 (112.05, -121.1912) -> (114.75, -119.6323)
  line L79 (114.75, -119.6323) -> (117.45, -121.1912)
  line L80 (159.75, -59.8677) -> (157.05, -58.3088)
  line L81 (157.05, -58.3088) -> (157.05, -55.1912)
  line L82 (157.05, -55.1912) -> (159.75, -53.6323)
  line L83 (159.75, -53.6323) -> (162.45, -55.1912)
  line L84 (162.45, -55.1912) -> (162.45, -58.3088)
  line L85 (162.45, -58.3088) -> (159.75, -59.8677)
  line L86 (117.45, -58.3088) -> (114.75, -59.8677)
  line L87 (114.75, -59.8677) -> (112.05, -58.3088)
  line L88 (112.05, -58.3088) -> (112.05, -55.1912)
  line L89 (112.05, -55.1912) -> (114.75, -53.6323)
  line L90 (114.75, -53.6323) -> (117.45, -55.1912)
  line L91 (117.45, -55.1912) -> (117.45, -58.3088)
  circle A44 centre (-114.25, 78.75) radius 5.11
  circle A45 centre (-114.25, -78.75) radius 5.11
  point P0 (-80, 0)
  point P1 (80, 0)
  point P2 (159.75, -122.75)
  dimension "d158" = 80
  dimension "d160" = 6
  dimension "d164" = 10.22
  dimension "d166" = 2
  dimension "d172" = 6
  dimension "d174" = 9.9
  dimension "d175" = 35
  dimension "d176" = 9.95
  dimension "d177" = 9.9
  dimension "d264" = 5.4
  dimension "d267" = 2
  dimension "d269" = 9.5
  dimension "d271" = 2
  dimension "d276" = 5.4
  dimension "d277" = 5.4
  dimension "d278" = 5.4
  constraints: 172 end point, 48 point on circle, 36 tangent, 34 centre point, 32 point on line, 30 symmetric about line, 22 coincident, 16 equal radius, 10 parallel, 9 midpoint, 8 vertical, 7 equal length, 5 horizontal, 4 perpendicular, 1 horizontal alignment, 89 other
  measures "d158" distance from line of L9 L12.start
  measures "d160" diameter of A10
  measures "d164" diameter of A12
  measures "d166" distance between parallel lines of L11 L19
  measures "d172" diameter of A11
  measures "d174" distance between parallel lines of L24 L21
  measures "d175" distance of L11.start L11.end
  measures "d176" radius of A9
  measures "d177" distance between parallel lines of L15 L18
  measures "d264" distance between parallel lines of L71 L68
  measures "d267" radius of A28
  measures "d269" distance of L60.end L61.end
  measures "d271" radius of A32
  measures "d276" distance between parallel lines of L77 L74
  measures "d277" distance between parallel lines of L81 L84
  measures "d278" distance between parallel lines of L88 L91
extrude "Выдавливание2" cut sketch "Эскиз2" against normal blind 8 contours L0 A0 L1 A1 | A1 | A0 | A2 | A2 L2 A3 L3 | A3 | A5 L5 A4 L4 | A5 | A4 | A6 L7 A7 L6 | A6 | A7
extrude "Выдавливание6" cut sketch "Эскиз2" against normal blind 4 contours A13 L25 L9 | L9 L26 A13 | A13 L26 L21 L22 L23 L24 L25 | A13 L26 | L25 A13 | L26 L21 A13 | A13 L24 L25 | A13 L21 | L24 A13 | L21 L22 A13 | A13 L23 L24 | A13 L22 | L23 A13 | L22 L23 A13 | L15 A12 L9 | L9 A12 L14 | A12 L15 L16 L17 L18 L13 L14 | L14 A12 | A12 L15 | A12 L13 L14 | L15 L16 A12 | L13 A12 | A12 L16 | A12 L18 L13 | L16 L17 A12 | L18 A12 | A12 L17 | A12 L17 L18 | A10 | A11 | A15 L20 A14 L19 | A16 | L32 A20 L27 | A20 L32 L30 L31 L29 L28 L27 | L27 A20 | A20 L32 | A20 L28 L27 | L32 L30 A20 | L28 A20 | A20 L30 | A20 L29 L28 | L30 L31 A20 | L29 A20 | A20 L31 | A20 L35 L29 | L31 L35 A20 | L34 A23 L36 A18 | A19 | A22 L43 L35 | L35 L42 A22 | A22 L42 L41 L40 L39 L38 L43 | A22 L42 | L43 A22 | L42 L41 A22 | A22 L38 L43 | A22 L41 | L38 A22 | L41 L40 A22 | A22 L39 L38 | A22 L40 | L39 A22 | L40 L39 A22
extrude "Выдавливание7" cut sketch "Эскиз2" against normal through all contours A13 L26 L21 L22 L23 L24 L25 | A13 L26 | L25 A13 | A13 L21 | L24 A13 | A13 L22 | L23 A13 | A12 L15 L16 L17 L18 L13 L14 | L14 A12 | A12 L15 | L13 A12 | A12 L16 | L18 A12 | A12 L17 | A10 | A11 | A16 | A20 L32 L30 L31 L29 L28 L27 | L27 A20 | A20 L32 | L28 A20 | A20 L30 | L29 A20 | A20 L31 | A19 | A22 L42 L41 L40 L39 L38 L43 | A22 L42 | L43 A22 | A22 L41 | L38 A22 | A22 L40 | L39 A22
ref_plane "РабПлоскость1" through (0, 0, 4) normal (0, 0, 1) x (1, 0, 0)
extrude "Выдавливание8" cut sketch "Эскиз2" against normal blind 2.5 contours A24 | A25 | A26 | A27 | L44 A29 L45 A31 L46 A28 L47 A30 | L50 A34 L51 A35 L52 A32 L53 A33 | L56 A36 L57 A37 L58 A38 L59 A39 | L62 A40 L63 A41 L64 A42 L65 A43 | L68 L69 L70 L71 L72 L73 | L74 L75 L76 L77 L78 L79 | L80 L81 L82 L83 L84 L85 | L86 L87 L88 L89 L90 L91
extrude "Выдавливание9" cut sketch "Эскиз2" against normal blind 6 contours A24 | A25 | A26 | A27